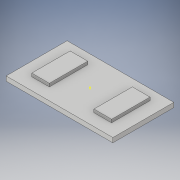
# Autodesk Inventor part: base explo
Saved by Autodesk Inventor 2019 (Build 230136000, 136)
## iProperties
Created: 2020-04-13
Part Number: base explo
Material: Generic
Document SubType Name: Modeling
Designer: DISHA PATIL
Density: 1 g/cm^3
Appearance: Default
Author: DISHA PATIL
Autodesk Inventor part; units mm, degrees
ref_plane "YZ Plane" through (0, 0, 0) normal (1, 0, 0) x (0, 1, 0)
ref_plane "XZ Plane" through (0, 0, 0) normal (0, 1, 0) x (-1, 0, 0)
ref_plane "XY Plane" through (0, 0, 0) normal (0, 0, 1) x (1, 0, 0)
sketch "Sketch1" plane through (0, 0, 0) normal (0, 1, 0) x (-1, 0, 0)
  point P0 (0, 0)
sketch "Sketch2" plane through (0, 0, 0) normal (0, 1, 0) x (-1, 0, 0)
  line L0 (175, 100) -> (-175, 100)
  line L1 (-175, 100) -> (-175, -100)
  line L2 (-175, -100) -> (175, -100)
  line L3 (175, -100) -> (175, 100)
  line L4 (175, -100) -> (-22.9318, -100)
  point P0 (0, 0)
  point P1 (0, -168.5892)
  point P2 (215.1093, 0)
  dimension "d0" = 350
  dimension "d1" = 200
  dimension "d4" = 175
  dimension "d5" = 100
  constraints: 10 end point, 2 parallel, 1 horizontal, 1 perpendicular, 1 point on line, 2 other
  measures "d0" distance of L2.end L1.end
  measures "d1" distance of L1.end L0.end
  measures "d4" distance from line of point (0, -168.589) L3
  measures "d5" distance from line of L2 point (215.109, 0)
extrude "Extrusion1" add sketch "Sketch2" along normal blind 15
sketch "Sketch3" plane through (0, 15, 0) normal (0, 1, 0) x (1, 0, 0)
  point P0 (0, 0)
sketch "Sketch4" plane through (0, 15, 0) normal (0, 1, 0) x (1, 0, 0)
  line L0 (-131.0663, -60.2343) -> (-73.0663, -60.2343)
  line L1 (-73.0663, -60.2343) -> (-73.0663, 65.7657)
  line L2 (-73.0663, 65.7657) -> (-131.0663, 65.7657)
  line L3 (-131.0663, 65.7657) -> (-131.0663, -60.2343)
  point P0 (0, 0)
  dimension "d6" = 58
  dimension "d7" = 126
  constraints: 8 end point, 2 parallel, 1 horizontal, 1 perpendicular
  measures "d6" distance of L2.end L1.end
  measures "d7" distance of L1.end L0.end
extrude "Extrusion2" add sketch "Sketch4" along normal blind 5
sketch "Sketch5" plane through (0, 15, 0) normal (0, 1, 0) x (1, 0, 0)
  line L0 (-73.0663, -60.2343) -> (-73.0663, 65.7657) projected
  line L1 (0, 0) -> (73.066, 0)
  line L2 (73.066, -60.2343) -> (131.066, -60.2343)
  line L3 (131.066, -60.2343) -> (131.066, 65.7657)
  line L4 (131.066, 65.7657) -> (73.066, 65.7657)
  line L5 (73.066, 65.7657) -> (73.066, -60.2343)
  dimension "d10" = 73.066
  dimension "d11" = 58
  dimension "d12" = 126
  constraints: 10 end point, 2 horizontal, 2 parallel, 1 perpendicular
  measures "d10" distance of L1.start L1.end
  measures "d11" distance of L4.end L3.end
  measures "d12" distance of L3.end L2.end
extrude "Extrusion3" add sketch "Sketch5" along normal blind 5
sketch "Sketch6" plane through (0, 20, 0) normal (0, 1, 0) x (1, 0, 0)
  line L0 (73.066, -60.2343) -> (131.066, -60.2343) projected
  line L1 (131.066, -60.2343) -> (131.066, 65.7657) projected
  line L2 (73.066, -60.2343) -> (131.066, -60.2343)
  line L3 (131.066, -60.2343) -> (131.066, 65.7657)
  line L4 (131.066, 65.7657) -> (73.066, 65.7657)
  line L5 (73.066, 65.7657) -> (73.066, -60.2343)
  point P0 (0, 0)
  constraints: 8 end point, 2 parallel, 1 horizontal, 1 perpendicular
sketch "Sketch7" plane through (0, 20, 0) normal (0, 1, 0) x (1, 0, 0)
  line L0 (-131.0663, -60.2343) -> (-131.0663, 65.7657) projected
  line L1 (-73.0663, -60.2343) -> (-73.0663, 65.7657) projected
  line L2 (-131.0663, -60.2343) -> (-73.0663, -60.2343)
  line L3 (-73.0663, -60.2343) -> (-73.0663, 65.7657)
  line L4 (-73.0663, 65.7657) -> (-131.0663, 65.7657)
  line L5 (-131.0663, 65.7657) -> (-131.0663, -60.2343)
  point P0 (0, 0)
  constraints: 8 end point, 2 parallel, 1 horizontal, 1 perpendicular
extrude "Extrusion4" add sketch "Sketch7" along normal blind 5
sketch "Sketch8" plane through (0, 20, 0) normal (0, 1, 0) x (1, 0, 0)
  point P0 (0, 0)
extrude "Extrusion5" add sketch "Sketch6" along normal blind 5
body "Solid1"
